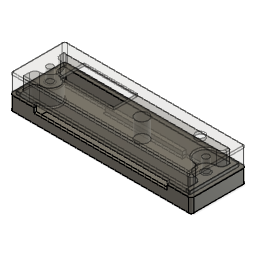
Keyboard Dongle Case (Autodesk Fusion 360 design; units mm, degrees)
part number: Bottom
part number: Top
Autodesk Fusion 360 part; units mm, degrees
sketch "Sketch1" plane through (0, 0, 0) normal (0, 1, 0) x (1, 0, 0)
  line L0 (0, 0) -> (65, 0)
  line L1 (65, 0) -> (65, -17.5)
  line L2 (65, -17.5) -> (0, -17.5)
  line L3 (0, -17.5) -> (0, 0)
  line L4 (-3, 3) -> (68, 3)
  line L5 (68, 3) -> (68, -18.5)
  line L6 (68, -18.5) -> (-3, -18.5)
  line L7 (-3, -18.5) -> (-3, 3)
  dimension "d3" = 71
  dimension "d4" = 21.5
  dimension "d5" = 3
  dimension "d6" = 3
  dimension "d41" = 3
  dimension "d42" = 1
  constraint horizontal L0
  constraint vertical L1
  constraint horizontal L2
  constraint vertical L3
  constraint coincident L0.start L3.end
  constraint horizontal L4
  constraint vertical L5
  constraint horizontal L6
  constraint vertical L7
  measures "d3" distance of L4.start L4.end
  measures "d4" distance of L4.start L6.end
  measures "d5" distance of L0 L4
  measures "d6" distance of L3 L7
  measures "d42" distance of L2 L6
extrude "Extrude1" add sketch "Sketch1" along normal blind 7 contours L0 L1 L2 L3 | L4 L5 L6 L7 makes body 1
sketch "Sketch2" plane through (0, 7, 0) normal (0, 1, 0) x (-1, 0, 0)
  line L0 (3, 18.5) -> (-68, 18.5)
  line L1 (-68, 18.5) -> (-68, -3)
  line L2 (-68, -3) -> (3, -3)
  line L3 (3, -3) -> (3, 18.5)
  line L4 (0, 0) -> (-65, 0)
  line L5 (-65, 0) -> (-65, 17.5)
  line L6 (-65, 17.5) -> (0, 17.5)
  line L7 (0, 17.5) -> (0, 0)
  dimension "d9" = 3
  dimension "d10" = 1
  dimension "d11" = 3
  dimension "d12" = 3
  constraint horizontal L4
  constraint vertical L5
  constraint horizontal L6
  constraint vertical L7
  measures "d9" distance of L2 L4
  measures "d10" distance of L0 L6
  measures "d11" distance of L1 L5
  measures "d12" distance of L3 L7
extrude "Extrude2" cut sketch "Sketch2" against normal blind 6 contours L4 L5 L6 L7 bodies 1
sketch "Sketch3" plane through (0, 1, 0) normal (0, 1, 0) x (-1, 0, 0)
  line L0 (0, 17.5) -> (-65, 17.5)
  line L1 (-65, 17.5) -> (-65, 0)
  line L2 (-65, 0) -> (0, 0)
  line L3 (0, 0) -> (0, 17.5)
  line L4 (-7.5, 14.5) -> (-57.5, 14.5)
  line L5 (-57.5, 14.5) -> (-57.5, 16.5)
  line L6 (-57.5, 16.5) -> (-7.5, 16.5)
  line L7 (-7.5, 16.5) -> (-7.5, 14.5)
  line L8 (-17.5, 0) -> (-47.5, 0)
  line L9 (-47.5, 0) -> (-47.5, 1.5)
  line L10 (-47.5, 1.5) -> (-17.5, 1.5)
  line L11 (-17.5, 1.5) -> (-17.5, 0)
  line L12 (-68, -3) -> (3, -3)
  circle A0 centre (-2, 7.25) radius 3.5
  circle A1 centre (-63, 7.25) radius 3.5
  line L13 (3, -3) -> (3, 18.5)
  line L14 (-68, 18.5) -> (-68, -3)
  line L15 (3, 18.5) -> (-68, 18.5)
  dimension "d17" = 2
  dimension "d18" = 1
  dimension "d21" = 30
  dimension "d22" = 1.5
  dimension "d24" = 20.5
  dimension "d26" = 3
  dimension "d27" = 50
  dimension "d28" = 10.5
  dimension "d29" = 7
  dimension "d30" = 7
  dimension "d31" = 5
  dimension "d32" = 5
  dimension "d33" = 20.5
  dimension "d34" = 10.25
  dimension "d35" = 10.25
  constraint horizontal L4
  constraint vertical L5
  constraint horizontal L6
  constraint vertical L7
  constraint horizontal L8
  constraint vertical L9
  constraint horizontal L10
  constraint vertical L11
  measures "d17" distance of L4 L6
  measures "d18" distance of L0 L6
  measures "d21" distance of L8.start L8.end
  measures "d22" distance of L8.start L10.end
  measures "d24" distance of L11 L12.end
  measures "d26" distance of L8 L12
  measures "d27" distance of L4.start L4.end
  measures "d28" distance of L7 L12.end
  measures "d29" diameter of A0
  measures "d30" diameter of A1
  measures "d31" distance of A0.centre L13
  measures "d32" distance of A1.centre L14
  measures "d34" distance of L12 A0.centre
  measures "d35" distance of L12 A1.centre
extrude "Extrude3" add sketch "Sketch3" along normal blind 2 contours L2 L8 L9 L10 L11 | L4 L5 L6 L7 bodies 1
sketch "Sketch4" plane through (0, 1, 0) normal (0, 1, 0) x (-1, 0, 0)
  line L0 (-17.5, 0) -> (0, 0)
  line L1 (0, 0) -> (0, 17.5)
  line L2 (0, 17.5) -> (-65, 17.5)
  line L3 (-65, 17.5) -> (-65, 0)
  line L4 (-7.5, 16.5) -> (-7.5, 14.5)
  line L5 (-7.5, 14.5) -> (-57.5, 14.5)
  line L6 (-57.5, 14.5) -> (-57.5, 16.5)
  line L7 (-57.5, 16.5) -> (-7.5, 16.5)
  circle A0 centre (-2, 7.75) radius 4
  circle A1 centre (-63, 7.75) radius 4
  line L8 (3, -3) -> (3, 18.5)
  line L9 (-68, 18.5) -> (-68, -3)
  line L10 (-68, -3) -> (3, -3)
  line L11 (-47.5, 0) -> (-47.5, 1.5)
  line L12 (-47.5, 1.5) -> (-17.5, 1.5)
  line L13 (-17.5, 1.5) -> (-17.5, 0)
  line L14 (-65, 0) -> (-47.5, 0)
  dimension "d43" = 8
  dimension "d44" = 8
  dimension "d45" = 5
  dimension "d46" = 5
  dimension "d47" = 10.75
  dimension "d48" = 10.75
  measures "d43" diameter of A0
  measures "d44" diameter of A1
  measures "d45" distance of A0.centre L8
  measures "d46" distance of A1.centre L9
  measures "d47" distance of A0.centre L10
  measures "d48" distance of A1.centre L10
extrude "Extrude4" add sketch "Sketch4" along normal up to surface (6 mm away) contours L1 A0 | L3 A1 picked at (-1.9851, 7.5513) picked at (-63.0592, 7.357) bodies 1
sketch "Sketch5" plane through (0, 7, 0) normal (0, 1, 0) x (-1, 0, 0)
  line L0 (-65, 0) -> (-65, 4.2859)
  arc A0 (-65, 4.2859) -> (-65, 11.2141) centre (-63, 7.75) ccw
  line L1 (-65, 11.2141) -> (-65, 17.5)
  line L2 (-65, 17.5) -> (0, 17.5)
  line L3 (0, 17.5) -> (0, 11.2141)
  arc A1 (0, 11.2141) -> (0, 4.2859) centre (-2, 7.75) ccw
  line L4 (0, 4.2859) -> (0, 0)
  line L5 (0, 0) -> (-65, 0)
  line L6 (3, 18.5) -> (-68, 18.5)
  line L7 (-68, 18.5) -> (-68, -3)
  line L8 (-68, -3) -> (3, -3)
  line L9 (3, -3) -> (3, 18.5)
  circle A2 centre (-2, 7.75) radius 1.75
  circle A3 centre (-63, 7.75) radius 1.75
  dimension "d51" = 3.5
  dimension "d52" = 3.5
  constraint concentric A1 A2
  constraint concentric A0 A3
  measures "d51" diameter of A2
  measures "d52" diameter of A3
extrude "Extrude5" cut sketch "Sketch5" against normal through all contours A2 | A3 bodies 1
fillet "Fillet1" radius 2 4 edges at (0, 4, 4.2859) (0, 4, 11.2141) (65, 4, 11.2141) (65, 4, 4.2859) on bodies 1
fillet "Fillet2" radius 0.5 1 faces at (37.5, 1, 10.1667) on bodies 1
fillet "Fillet3" radius 0.5 8 edges at (0, 4.25, 0) (0.1464, 1.1464, 0.1464) (65, 4.25, 0) (64.8536, 1.1464, 0.1464) (65, 4.25, 17.5) (64.8536, 1.1464, 17.3536) (0, 4.25, 17.5) (0.1464, 1.1464, 17.3536) on bodies 1
fillet "Fillet4" radius 1 4 edges at (68, 3.5, 18.5) (68, 3.5, -3) (-3, 3.5, 18.5) (-3, 3.5, -3) on bodies 1
sketch "Sketch7" plane through (0, 7, 0) normal (0, 1, 0) x (-1, 0, 0)
  arc A0 (2, -3) -> (3, -2) centre (2, -2) ccw
  line L0 (3, -2) -> (3, 17.5)
  arc A1 (3, 17.5) -> (2, 18.5) centre (2, 17.5) ccw
  line L1 (2, 18.5) -> (-67, 18.5)
  arc A2 (-67, 18.5) -> (-68, 17.5) centre (-67, 17.5) ccw
  line L2 (-68, 17.5) -> (-68, -2)
  arc A3 (-68, -2) -> (-67, -3) centre (-67, -2) ccw
  line L3 (-67, -3) -> (2, -3)
  circle A4 centre (-2, 7.75) radius 1.75
  circle A5 centre (-63, 7.75) radius 1.75
  line L4 (-65, 0.5) -> (-65, 1.75)
  arc A6 (-63, 3.75) -> (-65, 1.75) centre (-63, 1.75) ccw
  arc A7 (-63, 3.75) -> (-63, 11.75) centre (-63, 7.75) ccw
  arc A8 (-65, 13.75) -> (-63, 11.75) centre (-63, 13.75) ccw
  line L5 (-65, 13.75) -> (-65, 17)
  arc A9 (-64.5, 17.5) -> (-65, 17) centre (-64.5, 17) ccw
  line L6 (-64.5, 17.5) -> (-0.5, 17.5)
  arc A10 (0, 17) -> (-0.5, 17.5) centre (-0.5, 17) ccw
  line L7 (0, 17) -> (0, 13.75)
  arc A11 (-2, 11.75) -> (0, 13.75) centre (-2, 13.75) ccw
  arc A12 (-2, 11.75) -> (-2, 3.75) centre (-2, 7.75) ccw
  arc A13 (0, 1.75) -> (-2, 3.75) centre (-2, 1.75) ccw
  line L8 (0, 1.75) -> (0, 0.5)
  arc A14 (-0.5, 0) -> (0, 0.5) centre (-0.5, 0.5) ccw
  line L9 (-0.5, 0) -> (-64.5, 0)
  arc A15 (-65, 0.5) -> (-64.5, 0) centre (-64.5, 0.5) ccw
  line L10 (1.4005, -1.4005) -> (1.4005, 17.4)
  line L11 (-66.4005, 17.4) -> (-66.4005, -1.4005)
  line L12 (-66.4005, -1.4005) -> (1.4005, -1.4005)
  line L13 (3.0005, -2) -> (3.0005, 17.5)
  arc A16 (3.0005, 17.5) -> (2, 18.5005) centre (2, 17.5) ccw
  arc A17 (-66.9691, 18.5) -> (-68.0005, 17.5) centre (-67, 17.5) ccw
  line L14 (-68.0005, 17.5) -> (-68.0005, -2)
  arc A18 (-68.0005, -2) -> (-67, -3.0005) centre (-67, -2) ccw
  line L15 (-67, -3.0005) -> (2, -3.0005)
  arc A19 (2, -3.0005) -> (3.0005, -2) centre (2, -2) ccw
  line L16 (1.4005, 17.4) -> (1.4005, 18.5005)
  line L17 (2, 18.5005) -> (1.4005, 18.5005)
  line L18 (-66.4005, 17.4) -> (-66.4005, 18.5)
  line L19 (-66.9691, 18.5) -> (-66.4005, 18.5)
  dimension "d64" = 1.6
  dimension "d65" = 1.6
  dimension "d66" = 1.6
  constraint parallel L0 L10
  constraint parallel L2 L11
  constraint parallel L3 L12
  constraint parallel L0 L13
  constraint concentric A1 A16
  constraint concentric A2 A17
  constraint parallel L2 L14
  constraint concentric A3 A18
  constraint parallel L3 L15
  constraint concentric A0 A19
  constraint tangent L15 A19
  constraint tangent A17 L14
  constraint tangent L13 A19
  constraint tangent L13 A16
  constraint tangent L14 A18
  constraint tangent A18 L15
  constraint parallel L10 L16
  constraint tangent A16 L17
  constraint perpendicular L16 L17
  constraint parallel L11 L18
  constraint tangent A2 L19
  constraint parallel L1 L19
  measures "d64" distance of L10 L13
  measures "d65" distance of L12 L15
  measures "d66" distance of L11 L14
extrude "Extrude6" cut sketch "Sketch7" against normal blind 1.2 contours A0 L0 A1 L1 A2 L2 A3 L3 L10 L11 L12 L13 A16 A17 L14 A18 L15 A19 L16 L17 L18 L19 bodies 1
sketch "Sketch8" plane through (0, 7, 0) normal (0, 1, 0) x (-1, 0, 0)
  line L0 (1.4005, -1.4005) -> (1.4005, 18.5)
  line L1 (1.4005, 18.5) -> (-66.4005, 18.5)
  line L2 (-66.4005, 18.5) -> (-66.4005, -1.4005)
  line L3 (-66.4005, -1.4005) -> (1.4005, -1.4005)
  circle A0 centre (-2, 7.75) radius 1.75
  circle A1 centre (-63, 7.75) radius 1.75
  line L4 (-65, 0.5) -> (-65, 1.75)
  arc A2 (-63, 3.75) -> (-65, 1.75) centre (-63, 1.75) ccw
  arc A3 (-63, 3.75) -> (-63, 11.75) centre (-63, 7.75) ccw
  arc A4 (-65, 13.75) -> (-63, 11.75) centre (-63, 13.75) ccw
  line L5 (-65, 13.75) -> (-65, 17)
  arc A5 (-64.5, 17.5) -> (-65, 17) centre (-64.5, 17) ccw
  line L6 (-64.5, 17.5) -> (-0.5, 17.5)
  arc A6 (0, 17) -> (-0.5, 17.5) centre (-0.5, 17) ccw
  line L7 (0, 17) -> (0, 13.75)
  arc A7 (-2, 11.75) -> (0, 13.75) centre (-2, 13.75) ccw
  arc A8 (-2, 11.75) -> (-2, 3.75) centre (-2, 7.75) ccw
  arc A9 (0, 1.75) -> (-2, 3.75) centre (-2, 1.75) ccw
  line L8 (0, 1.75) -> (0, 0.5)
  arc A10 (-0.5, 0) -> (0, 0.5) centre (-0.5, 0.5) ccw
  line L9 (-0.5, 0) -> (-64.5, 0)
  arc A11 (-65, 0.5) -> (-64.5, 0) centre (-64.5, 0.5) ccw
  line L10 (-6.5, 17.5) -> (-58.5, 17.5)
  line L11 (-58.5, 17.5) -> (-58.5, 18.5)
  line L12 (-58.5, 18.5) -> (-6.5, 18.5)
  line L13 (-6.5, 18.5) -> (-6.5, 17.5)
  line L14 (-68, -2) -> (-68, 17.5)
  dimension "d69" = 52
  dimension "d70" = 9.5
  constraint horizontal L10
  constraint vertical L11
  constraint horizontal L12
  constraint vertical L13
  constraint coincident L1 L11.end
  constraint coincident L6 L10.start
  measures "d69" distance of L11.end L12.end
  measures "d70" distance of L11.end L14
extrude "Extrude7" cut sketch "Sketch8" against normal blind 3 contours L1 L6 L10 L11 L12 L13 bodies 1
ref_plane "WorkPlane1" through (32.5, 13.2, 7.75) normal (0, 1, 0) x (0, 0, 1)
sketch "Sketch10" plane through (33, 13.2, 8.85) normal (0, 1, 0) x (1, 0, 0)
  arc A0 (-36, 10.85) -> (-35, 11.85) centre (-35, 10.85) cw
  line L0 (-36, -8.65) -> (-36, 10.85)
  arc A1 (-35, -9.65) -> (-36, -8.65) centre (-35, -8.65) cw
  line L1 (-34.4005, -9.65) -> (-35, -9.65)
  line L2 (-34.4005, -9.65) -> (-26.5, -9.65)
  line L3 (25.5, -9.65) -> (-26.5, -9.65)
  line L4 (25.5, -9.65) -> (33.4005, -9.65)
  line L5 (34, -9.65) -> (33.4005, -9.65)
  arc A2 (35, -8.65) -> (34, -9.65) centre (34, -8.65) cw
  line L6 (35, 10.85) -> (35, -8.65)
  arc A3 (34, 11.85) -> (35, 10.85) centre (34, 10.85) cw
  line L7 (-35, 11.85) -> (34, 11.85)
extrude "Extrude8" add sketch "Sketch10" against normal blind 6 separate body makes body 2
sketch "Sketch12" plane through (0, 7.2, 0) normal (0, -1, 0) x (1, 0, 0)
  line L0 (0, 15) -> (0, 0)
  line L1 (0, 0) -> (65, 0)
  line L2 (65, 0) -> (65, 14.5)
  line L3 (0, 15) -> (0, 16.5)
  line L4 (65, 14.5) -> (65, 16.5)
  line L5 (0, 16.5) -> (65, 16.5)
  line L6 (67, 18.5) -> (-2, 18.5)
  arc A0 (-2, 18.5) -> (-3, 17.5) centre (-2, 17.5) ccw
  line L7 (-3, 17.5) -> (-3, -2)
  arc A1 (-3, -2) -> (-2, -3) centre (-2, -2) ccw
  line L8 (-2, -3) -> (67, -3)
  arc A2 (67, -3) -> (68, -2) centre (67, -2) ccw
  line L9 (68, -2) -> (68, 17.5)
  arc A3 (68, 17.5) -> (67, 18.5) centre (67, 17.5) ccw
  constraint perpendicular L3 L5
  constraint parallel L2 L4
extrude "Extrude9" cut sketch "Sketch12" against normal blind 5 contours L0 L1 L2 L3 L4 L5 bodies 2
sketch "Sketch15" plane through (0, 7.2, 0) normal (0, -1, 0) x (1, 0, 0)
  line L0 (67, 18.5) -> (-2, 18.5)
  arc A0 (-2, 18.5) -> (-3, 17.5) centre (-2, 17.5) ccw
  line L1 (-3, 17.5) -> (-3, -2)
  arc A1 (-3, -2) -> (-2, -3) centre (-2, -2) ccw
  line L2 (-2, -3) -> (67, -3)
  arc A2 (67, -3) -> (68, -2) centre (67, -2) ccw
  line L3 (68, -2) -> (68, 17.5)
  arc A3 (68, 17.5) -> (67, 18.5) centre (67, 17.5) ccw
  line L4 (-1.6, 17.5) -> (66.6, 17.5)
  line L5 (66.6, 17.5) -> (66.6, -1.6)
  line L6 (66.6, -1.6) -> (-1.6, -1.6)
  line L7 (-1.6, -1.6) -> (-1.6, 17.5)
  dimension "d141" = 1.4
  dimension "d142" = 1.4
  dimension "d143" = 1.4
  dimension "d144" = 1
  constraint horizontal L4
  constraint vertical L5
  constraint horizontal L6
  constraint vertical L7
  measures "d141" distance of L1 L7
  measures "d142" distance of L3 L5.end
  measures "d143" distance of L2 L6
  measures "d144" distance of L0 L4
extrude "Extrude11" add sketch "Sketch15" along normal blind 1.2 bodies 2
sketch "Sketch17" plane through (0, 7, 0) normal (0, 1, 0) x (-1, 0, 0)
  circle A0 centre (-63, 7.75) radius 1.75
  circle A1 centre (-2, 7.75) radius 1.75
  line L0 (-58.5, 17.5) -> (-58.5, 18.5)
  line L1 (-58.5, 18.5) -> (-66.4005, 18.5)
  line L2 (-66.4005, 18.5) -> (-66.4005, -1.4005)
  line L3 (-66.4005, -1.4005) -> (1.4005, -1.4005)
  line L4 (1.4005, -1.4005) -> (1.4005, 18.5)
  line L5 (1.4005, 18.5) -> (-6.5, 18.5)
  line L6 (-6.5, 18.5) -> (-6.5, 17.5)
  line L7 (-6.5, 17.5) -> (-0.5, 17.5)
  arc A2 (0, 17) -> (-0.5, 17.5) centre (-0.5, 17) ccw
  line L8 (0, 17) -> (0, 13.75)
  arc A3 (-2, 11.75) -> (0, 13.75) centre (-2, 13.75) ccw
  arc A4 (-2, 11.75) -> (-2, 3.75) centre (-2, 7.75) ccw
  arc A5 (0, 1.75) -> (-2, 3.75) centre (-2, 1.75) ccw
  line L9 (0, 1.75) -> (0, 0.5)
  arc A6 (-0.5, 0) -> (0, 0.5) centre (-0.5, 0.5) ccw
  line L10 (-0.5, 0) -> (-64.5, 0)
  arc A7 (-65, 0.5) -> (-64.5, 0) centre (-64.5, 0.5) ccw
  line L11 (-65, 0.5) -> (-65, 1.75)
  arc A8 (-63, 3.75) -> (-65, 1.75) centre (-63, 1.75) ccw
  arc A9 (-63, 3.75) -> (-63, 11.75) centre (-63, 7.75) ccw
  arc A10 (-65, 13.75) -> (-63, 11.75) centre (-63, 13.75) ccw
  line L12 (-65, 13.75) -> (-65, 17)
  arc A11 (-64.5, 17.5) -> (-65, 17) centre (-64.5, 17) ccw
  line L13 (-64.5, 17.5) -> (-58.5, 17.5)
  line L14 (1.4005, 17.5) -> (1.4005, 18.5)
  line L15 (1.4005, 18.5) -> (-6.5, 18.5)
  line L16 (-6.5, 18.5) -> (-6.5, 17.5)
  line L17 (-66.4005, 17.5) -> (-66.4005, 18.5)
  line L18 (-66.4005, 18.5) -> (-58.5, 18.5)
  line L19 (-58.5, 18.5) -> (-58.5, 17.5)
  line L20 (-65, 17) -> (-65, 17.5)
  line L21 (-64.5, 17.5) -> (-64.5, 17)
  line L22 (-64.5, 17) -> (-65, 17)
  line L23 (-58.5, 17.5) -> (-64.5, 17.5)
  line L24 (-65, 17.5) -> (-66.4005, 17.5)
  line L25 (0, 17) -> (0, 17.5)
  line L26 (-0.5, 17.5) -> (-0.5, 17)
  line L27 (-0.5, 17) -> (0, 17)
  line L28 (-6.5, 17.5) -> (-0.5, 17.5)
  line L29 (0, 17.5) -> (1.4005, 17.5)
  constraint horizontal L28
  constraint vertical L14
  constraint horizontal L15
  constraint vertical L16
  constraint coincident L4.end L5.start
  constraint coincident L6.end L7.start
  constraint horizontal L23
  constraint vertical L17
  constraint horizontal L18
  constraint vertical L19
  constraint coincident L1.end L2.start
  constraint coincident L0.start L13.end
  constraint coincident L12.end A11.end
  constraint coincident L20.end L23
  constraint tangent A11 L20
  constraint coincident A11.start L13.start
  constraint coincident A11.centre L21.end
  constraint collinear L23 L24
  constraint coincident A2.start L8.start
  constraint coincident L25.end L28
  constraint tangent A2 L25
  constraint coincident L7.end A2.end
  constraint coincident A2.centre L26.end
  constraint collinear L28 L29
extrude "Extrude13" cut sketch "Sketch17" against normal up to surface (1.2 mm away) contours L0 L1 L2 A11 L13 L17 L18 L19 L20 L23 L24 | A11 L21 L22 | L4 L5 L6 L7 A2 L14 L15 L16 L25 L28 L29 | A2 L26 L27 bodies 1
sketch "Sketch18" plane through (0, 0, 18.5) normal (0, 0, 1) x (1, 0, 0)
  line L0 (6.5, 6) -> (58.5, 6)
  line L1 (58.5, 6) -> (58.5, 7)
  line L2 (58.5, 7) -> (6.5, 7)
  line L3 (6.5, 7) -> (6.5, 6)
  line L4 (68, 13.2) -> (68, 6)
  line L5 (-3, 13.2) -> (-3, 6)
  line L6 (67, 13.2) -> (-2, 13.2)
  line L7 (-2, 13.2) -> (-2, 6)
  line L8 (-2, 6) -> (67, 6)
  line L9 (67, 6) -> (67, 13.2)
  dimension "d147" = 52
  dimension "d148" = 1
  dimension "d149" = 9.5
  constraint horizontal L0
  constraint vertical L1
  constraint horizontal L2
  constraint vertical L3
  measures "d147" distance of L0.start L0.end
  measures "d148" distance of L0 L2
  measures "d149" distance of L3 L5
extrude "Extrude14" cut sketch "Sketch18" against normal blind 3 contours L0 L1 L2 L3 L8 bodies 2
copy_body "Body->Comp1" bodies 1 removing the originals makes body 3 in component "Bottom"
copy_body "Body->Comp2" bodies 2 removing the originals makes body 4 in component "Top"
sketch "Sketch19" plane through (0, 13.2, 0) normal (0, 1, 0) x (-1, 0, 0)
  line L0 (-8.5, 0.9) -> (-29.25, 0.9)
  line L1 (-29.25, 0.9) -> (-29.25, 10.1)
  line L2 (-29.25, 10.1) -> (-8.5, 10.1)
  line L3 (-8.5, 10.1) -> (-8.5, 0.9)
  circle A0 centre (-55.5, 2.5) radius 1.75
  line L4 (2, 18.5) -> (-67, 18.5)
  arc A1 (-67, 18.5) -> (-68, 17.5) centre (-67, 17.5) ccw
  line L5 (-68, 17.5) -> (-68, -2)
  arc A2 (-68, -2) -> (-67, -3) centre (-67, -2) ccw
  line L6 (-67, -3) -> (2, -3)
  arc A3 (2, -3) -> (3, -2) centre (2, -2) ccw
  line L7 (3, -2) -> (3, 17.5)
  arc A4 (3, 17.5) -> (2, 18.5) centre (2, 17.5) ccw
  dimension "d95" = 20.75
  dimension "d96" = 9.2
  dimension "d99" = 3.5
  constraint horizontal L0
  constraint vertical L1
  constraint horizontal L2
  constraint vertical L3
  measures "d95" distance of L0.start L0.end
  measures "d96" distance of L0.start L2.end
  measures "d99" diameter of A0
extrude "Extrude1'" cut sketch "Sketch19" against normal blind 1 contours L0 L1 L2 L3 | A0 bodies 4 in component "Top"
sketch "Sketch20" plane through (0, 0, 0) normal (0, -1, 0) x (1, 0, 0)
  circle A0 centre (2, 7.75) radius 1.75
  circle A1 centre (63, 7.75) radius 1.75
  arc A2 (-3, -2) -> (-2, -3) centre (-2, -2) ccw
  line L0 (-2, -3) -> (67, -3)
  arc A3 (67, -3) -> (68, -2) centre (67, -2) ccw
  line L1 (68, -2) -> (68, 17.5)
  arc A4 (68, 17.5) -> (67, 18.5) centre (67, 17.5) ccw
  line L2 (67, 18.5) -> (-2, 18.5)
  arc A5 (-2, 18.5) -> (-3, 17.5) centre (-2, 17.5) ccw
  line L3 (-3, 17.5) -> (-3, -2)
  circle A6 centre (2, 7.75) radius 3
  circle A7 centre (63, 7.75) radius 3
  dimension "d104" = 6
  dimension "d105" = 6
  constraint concentric A0 A6
  constraint concentric A1 A7
  measures "d104" diameter of A6
  measures "d105" diameter of A7
extrude "Extrude1''" cut sketch "Sketch20" against normal blind 2 contours A6 | A7 bodies 3 in component "Bottom"
sketch "Sketch21" plane through (0, 12.2, 0) normal (0, -1, 0) x (1, 0, 0)
  line L0 (29.25, 10.1) -> (29.25, 0.9)
  line L1 (8.5, 0.9) -> (8.5, 10.1)
  line L2 (8.5, 10.1) -> (29.25, 10.1)
  line L3 (0, 16.5) -> (0, 0)
  line L4 (0, 0) -> (65, 0)
  line L5 (65, 0) -> (65, 16.5)
  arc A0 (2, 3.75) -> (2, 11.75) centre (2, 7.75) ccw
  circle A1 centre (63, 7.75) radius 1.25
  circle A2 centre (2, 7.75) radius 1.25
  circle A3 centre (2, 7.75) radius 4
  line L6 (-2, -3) -> (67, -3)
  line L7 (-3, 17.5) -> (-3, -2)
  line L8 (68, -2) -> (68, 17.5)
  circle A4 centre (63, 7.75) radius 4
  line L9 (29.25, 0.9) -> (8.5, 0.9)
  line L10 (65, 16.5) -> (0, 16.5)
  circle A5 centre (2, 7.75) radius 1.75
  dimension "d108" = 2.5
  dimension "d109" = 2.5
  dimension "d121" = 10.75
  dimension "d122" = 10.75
  dimension "d123" = 5
  dimension "d124" = 5
  dimension "d125" = 5
  dimension "d127" = 10.75
  dimension "d128" = 5
  constraint concentric A1 A4
  measures "d108" diameter of A1
  measures "d109" diameter of A2
  measures "d121" distance of A0.centre L6
  measures "d122" distance of A0.centre L6
  measures "d123" distance of A0.centre L7
  measures "d124" distance of A0.centre L7
  measures "d125" distance of A0.centre L7
  measures "d127" distance of A1.centre L6
  measures "d128" distance of A1.centre L8
extrude "Extrude2'" add sketch "Sketch21" along normal up to surface (5 mm away) contours L3 A0 A3 | L5 A4 | L5 A4 | A5 bodies 4 in component "Top"
sketch "Sketch22" plane through (0, 12.2, 0) normal (0, -1, 0) x (1, 0, 0)
  circle A0 centre (37, 6.75) radius 2.5
  line L0 (-3, 16.5) -> (-3, -2)
  line L1 (6.5, 17.5) -> (58.5, 17.5)
  line L2 (65, 0) -> (65, 4.2859)
  arc A1 (65, 11.2141) -> (65, 4.2859) centre (63, 7.75) ccw
  line L3 (0, 4.2859) -> (0, 0)
  arc A2 (0, 4.2859) -> (0, 11.2141) centre (2, 7.75) ccw
  line L4 (8.5, 0.9) -> (8.5, 10.1)
  line L5 (8.5, 10.1) -> (29.25, 10.1)
  line L6 (29.25, 10.1) -> (29.25, 0.9)
  line L7 (0, 0) -> (65, 0)
  line L8 (0, 16.5) -> (0, 11.2141)
  line L9 (29.25, 0.9) -> (8.5, 0.9)
  circle A3 centre (55.5, 2.5) radius 1.75
  line L10 (65, 11.2141) -> (65, 16.5)
  line L11 (65, 16.5) -> (0, 16.5)
  circle A4 centre (55.5, 2.5) radius 1.75
  line L12 (29.25, 10.1) -> (29.25, 0.9)
  line L13 (29.25, 0.9) -> (8.5, 0.9)
  line L14 (8.5, 0.9) -> (8.5, 10.1)
  line L15 (8.5, 10.1) -> (29.25, 10.1)
  arc A5 (0, 4.2859) -> (0, 11.2141) centre (2, 7.75) ccw
  line L16 (0, 4.2859) -> (0, 0)
  line L17 (0, 0) -> (65, 0)
  line L18 (65, 0) -> (65, 4.2859)
  arc A6 (65, 11.2141) -> (65, 4.2859) centre (63, 7.75) ccw
  line L19 (65, 11.2141) -> (65, 16.5)
  line L20 (65, 16.5) -> (0, 16.5)
  line L21 (0, 16.5) -> (0, 11.2141)
  dimension "d116" = 5
  dimension "d117" = 40
  dimension "d118" = 10.75
  measures "d116" diameter of A0
  measures "d117" distance of A0.centre L0
  measures "d118" distance of A0.centre L1
extrude "Extrude3'" add sketch "Sketch22" along normal blind 7.5 contours A0 bodies 4 in component "Top"
fillet "Fillet4'" radius 2 4 edges at (0, 9.7, 4.2859) (0, 9.7, 11.2141) (65, 9.7, 4.2859) (65, 9.7, 11.2141) on bodies 4 in component "Top"
fillet "Fillet6" radius 0.5 16 edges at (32.5, 12.2, 16.5) (65, 12.2, 0.875) (64.4142, 12.2, 3.1642) (59, 12.2, 7.75) (64.4142, 12.2, 12.3358) (65, 12.2, 15.125) (65, 9.7, 16.5) (0, 7.2, 15.125) (0.5858, 7.2, 12.3358) (6, 7.2, 7.75) (0.5858, 7.2, 3.1642) (0, 7.2, 0.875) (0, 9.7, 16.5) (0, 9.7, 0) (32.5, 12.2, 0) (65, 9.7, 0) on bodies 4 in component "Top"
fillet "Fillet1'" radius 0.5 8 edges at (-2.7071, 0, 18.2071) (-3, 0, 7.75) (-2.7071, 0, -2.7071) (32.5, 0, -3) (67.7071, 0, -2.7071) (68, 0, 7.75) (67.7071, 0, 18.2071) (32.5, 0, 18.5) on bodies 3 in component "Bottom"
fillet "Fillet7" radius 0.5 8 edges at (67.7071, 13.2, 18.2071) (68, 13.2, 7.75) (67.7071, 13.2, -2.7071) (32.5, 13.2, -3) (-2.7071, 13.2, -2.7071) (-3, 13.2, 7.75) (-2.7071, 13.2, 18.2071) (32.5, 13.2, 18.5) on bodies 4 in component "Top"
component "Bottom" placed x (1, 0, 0) y (0, 1, 0) z (0, 0, 1) at (0, 0, 0)
component "Top" placed x (1, 0, 0) y (0, 1, 0) z (0, 0, 1) at (0, 0, 0)
equation "d3 = Case_Width"
equation "d4 = Case_Height"
equation "d5 = Top_Wall"
equation "d6 = Side_Wall"
equation "d7 = Bottom_Case_Height"
equation "d9 = Top_Wall"
equation "d10 = Bottom_Wall"
equation "d11 = Side_Wall"
equation "d12 = Side_Wall"
equation "d13 = -( Bottom_Case_Height - Outer_Wall )"
equation "d24 = ( Case_Width - d21 ) / 2"
equation "d26 = Top_Wall"
equation "d28 = ( Case_Width - d27 ) / 2"
equation "d30 = d29"
equation "d32 = d31"
equation "d35 = d34"
equation "Case_Width = 71 mm"
equation "Case_Height = 21.5 mm"
equation "Side_Wall = 3 mm"
equation "Top_Wall = 3 mm"
equation "Bottom_Wall = 1 mm"
equation "d41 = Side_Wall"
equation "d42 = Bottom_Wall"
equation "d44 = d43"
equation "d46 = d45"
equation "d47 = ( Case_Height / 2 )"
equation "d48 = Case_Height / 2"
equation "d52 = d51"
equation "d62 = -Lip_Height"
equation "d65 = d64"
equation "d66 = d64"
equation "Bottom_Case_Height = 7 mm"
equation "Outer_Wall = 1 mm"
equation "d70 = ( Case_Width - d69 ) / 2"
equation "Top_Case_Height = 6 mm"
equation "d74 = Top_Case_Height + 0.2 mm"
equation "d75 = -Top_Case_Height"
equation "d79 = -( Top_Case_Height - Outer_Wall )"
equation "Lip_Height = 1.2 mm"
equation "d86 = Lip_Height"
equation "d93 = -Side_Wall"
equation "d102 = -Outer_Wall"
equation "d108 = d109"
equation "d118 = Case_Height / 2"
equation "d121 = Case_Height / 2"
equation "d122 = Case_Height / 2"
equation "d127 = d121"
equation "d137 = 1.40 mm"
equation "d138 = d137"
equation "d149 = ( Case_Width - d147 ) / 2"
